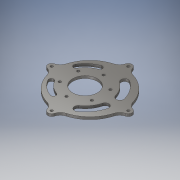
# Autodesk Inventor part: LargeBearingPlate
Saved by Autodesk Inventor 2019 (Build 230136000, 136)
## iProperties
Created: 2018-12-06
Part Number: LargeBearingPlate
Material: Aluminum 6061
Document SubType Name: Modeling
Designer: steelen
Density: 2.7 g/cm^3
Appearance: Semi-Polished
Author: steelen
Autodesk Inventor part; units mm, degrees
ref_plane "YZ Plane" through (0, 0, 0) normal (1, 0, 0) x (0, 1, 0)
ref_plane "XZ Plane" through (0, 0, 0) normal (0, 1, 0) x (-1, 0, 0)
ref_plane "XY Plane" through (0, 0, 0) normal (0, 0, 1) x (1, 0, 0)
sketch "Sketch1" plane through (0, 0, 0) normal (0, 1, 0) x (-1, 0, 0)
  circle A0 centre (12.7, 0) radius 31.75
  circle A1 centre (0, 0) radius 88.9
  circle A2 centre (0, 98.425) radius 9.525
  arc A3 (9.1574, 101.0457) -> (24.7665, 85.3805) centre (31.1351, 107.3355) ccw
  arc A4 (-24.7665, 85.3805) -> (-9.1574, 101.0457) centre (-31.1351, 107.3355) ccw
  circle A5 centre (-98.425, 0) radius 9.525
  circle A6 centre (0, -98.425) radius 9.525
  circle A7 centre (98.425, 0) radius 9.525
  arc A8 (85.3805, 24.7665) -> (101.0457, 9.1574) centre (107.3355, 31.1351) ccw
  arc A9 (24.7665, -85.3805) -> (9.1574, -101.0457) centre (31.1351, -107.3355) ccw
  arc A10 (-9.1574, -101.0457) -> (-24.7665, -85.3805) centre (-31.1351, -107.3355) ccw
  arc A11 (-85.3805, -24.7665) -> (-101.0457, -9.1574) centre (-107.3355, -31.1351) ccw
  arc A12 (-101.0457, 9.1574) -> (-85.3805, 24.7665) centre (-107.3355, 31.1351) ccw
  arc A13 (101.0457, -9.1574) -> (85.3805, -24.7665) centre (107.3355, -31.1351) ccw
  line L0 (98.425, 0) -> (88.9, 0)
  line L1 (0, 98.425) -> (0, 88.9)
  line L2 (0, -98.425) -> (0, -88.9)
  line L3 (-98.425, 0) -> (-88.9, 0)
  line L4 (12.7, 0) -> (0, 0)
  dimension "d20" = 177.8
  dimension "d0" = 63.5
  dimension "d2" = 19.05
  dimension "d3" = 22.86
  dimension "d21" = 12.7
  constraints: 27 point on circle, 13 centre point, 10 end point, 10 equal radius, 8 tangent, 3 horizontal, 3 vertical, 1 coincident, 26 other
  measures "d0" diameter of A0
  measures "d2" diameter of A2
  measures "d3" radius of A10
  measures "d21" distance of L4.start point (0, 0)
extrude "Extrusion1" add sketch "Sketch1" along normal blind 6.35
sketch "Sketch3" plane through (0, 6.35, 0) normal (0, 1, 0) x (1, 0, 0)
  circle A0 centre (-12.7, 0) radius 31.75 projected
  arc A1 (101.0457, -9.1574) -> (101.0457, 9.1574) centre (98.425, 0) ccw projected
  arc A2 (101.0457, -9.1574) -> (85.3805, -24.7665) centre (107.3355, -31.1351) ccw projected
  arc A3 (24.7665, -85.3805) -> (85.3805, -24.7665) centre (0, 0) ccw projected
  arc A4 (24.7665, -85.3805) -> (9.1574, -101.0457) centre (31.1351, -107.3355) ccw projected
  arc A5 (-9.1574, -101.0457) -> (9.1574, -101.0457) centre (0, -98.425) ccw projected
  arc A6 (-9.1574, -101.0457) -> (-24.7665, -85.3805) centre (-31.1351, -107.3355) ccw projected
  arc A7 (-85.3805, -24.7665) -> (-24.7665, -85.3805) centre (0, 0) ccw projected
  arc A8 (-85.3805, -24.7665) -> (-101.0457, -9.1574) centre (-107.3355, -31.1351) ccw projected
  arc A9 (-101.0457, 9.1574) -> (-101.0457, -9.1574) centre (-98.425, 0) ccw projected
  arc A10 (-101.0457, 9.1574) -> (-85.3805, 24.7665) centre (-107.3355, 31.1351) ccw projected
  arc A11 (-24.7665, 85.3805) -> (-85.3805, 24.7665) centre (0, 0) ccw projected
  arc A12 (-24.7665, 85.3805) -> (-9.1574, 101.0457) centre (-31.1351, 107.3355) ccw projected
  arc A13 (9.1574, 101.0457) -> (-9.1574, 101.0457) centre (0, 98.425) ccw projected
  arc A14 (9.1574, 101.0457) -> (24.7665, 85.3805) centre (31.1351, 107.3355) ccw projected
  arc A15 (85.3805, 24.7665) -> (24.7665, 85.3805) centre (0, 0) ccw projected
  arc A16 (85.3805, 24.7665) -> (101.0457, 9.1574) centre (107.3355, 31.1351) ccw projected
  constraints: 4 coincident
hole "Hole1" at (98.425, 6.35, 0) at (0, 6.35, 98.425) at (-98.425, 6.35, 0) at (0, 6.35, -98.425) direction (0, -1, 0) diameter 6.5278 depth 12.2936 tip angle 118 clearance for "Socket Head Cap Screw" size "1/4" standard "Ansi Unified Screw Threads"
sketch "Sketch8" plane through (0, 6.35, 0) normal (0, 1, 0) x (1, 0, 0)
  circle A0 centre (-12.7, 0) radius 31.75 projected
  circle A1 centre (-12.7, 0) radius 47.625
  line L0 (-12.7, 0) -> (-12.7, 47.625)
  point P0 (0, 0)
  point P1 (-53.9445, 23.8125)
  point P2 (-53.9445, -23.8125)
  point P3 (-12.7, -47.625)
  point P4 (28.5445, -23.8125)
  point P5 (28.5445, 23.8125)
  dimension "d38" = 95.25
  dimension "d41" = 360
  constraints: 2 end point, 1 coincident, 1 vertical, 1 vertical alignment, 9 other
hole "Hole3" at (-12.7, 6.35, -47.625) at (-53.9445, 6.35, -23.8125) at (-53.9445, 6.35, 23.8125) at (-12.7, 6.35, 47.625) at (28.5445, 6.35, 23.8125) at (28.5445, 6.35, -23.8125) direction (0, -1, 0) diameter 6.5278 end through all clearance for "Socket Head Cap Screw" size "1/4" standard "Ansi Unified Screw Threads"
sketch "Sketch9" plane through (0, 6.35, 0) normal (0, 1, 0) x (1, 0, 0)
  circle A0 centre (-12.7, 0) radius 31.75 projected
  circle A1 centre (-12.7, 0) radius 63.5
  circle A2 centre (-12.7, 0) radius 82.55
  arc A3 (34.6487, 67.621) -> (23.7221, 52.0162) centre (29.1854, 59.8186) ccw
  arc A4 (23.7221, -52.0162) -> (34.6487, -67.621) centre (29.1854, -59.8186) ccw
  line L0 (0, 0) -> (50.8, 0)
  line L1 (-12.7, 0) -> (29.1854, 59.8186)
  line L2 (29.1854, -59.8186) -> (-12.7, 0)
  arc A5 (67.0372, -21.3655) -> (48.6363, -16.435) centre (57.8367, -18.9003) ccw
  arc A6 (48.6363, 16.435) -> (67.0372, 21.3655) centre (57.8367, 18.9003) ccw
  line L3 (-12.7, 0) -> (57.8367, 18.9003)
  line L4 (-12.7, 0) -> (57.8367, -18.9003)
  dimension "d50" = 31.75
  dimension "d51" = 19.05
  dimension "d52" = 55
  dimension "d53" = 55
  dimension "d54" = 40
  dimension "d55" = 40
  constraints: 17 point on circle, 10 end point, 8 tangent, 6 centre point, 3 coincident, 1 horizontal
  measures "d50" radial gap between concentric circles of A1 A0
  measures "d51" radial gap between concentric circles of A1 A2
  measures "d52" angle of L2 L0
  measures "d53" angle of L0 L1
  measures "d54" angle of L1 L3
  measures "d55" angle of L2 L4
extrude "Extrusion3" cut sketch "Sketch9" against normal blind 25.4 contours A1 A3 A2 A6 | A5 A2 A4 A1
sketch "Sketch10" plane through (0, 6.35, 0) normal (0, 1, 0) x (1, 0, 0)
  circle A0 centre (-98.425, 0) radius 3.2639
  line L0 (-12.7, 0) -> (-98.425, 0)
  arc A1 (-32.2465, 53.7034) -> (-62.1934, 28.575) centre (-12.7, 0) ccw
  arc A2 (-73.1919, 34.925) -> (-62.1934, 28.575) centre (-67.6926, 31.75) ccw
  arc A3 (-32.2465, 53.7034) -> (-36.5901, 65.6375) centre (-34.4183, 59.6705) ccw
  arc A4 (-36.5901, 65.6375) -> (-73.1919, 34.925) centre (-12.7, 0) ccw
  circle A5 centre (-98.425, 0) radius 3.2639 projected
  circle A6 centre (-12.7, 0) radius 31.75 projected
  arc A7 (-62.1934, -28.575) -> (-32.2465, -53.7034) centre (-12.7, 0) ccw
  arc A8 (-62.1934, -28.575) -> (-73.1919, -34.925) centre (-67.6926, -31.75) ccw
  arc A9 (-36.5901, -65.6375) -> (-32.2465, -53.7034) centre (-34.4183, -59.6705) ccw
  arc A10 (-73.1919, -34.925) -> (-36.5901, -65.6375) centre (-12.7, 0) ccw
  circle A11 centre (-12.7, 0) radius 31.75
  dimension "d58" = 114.3
  dimension "d59" = 12.7
  dimension "d60" = 70
  dimension "d61" = 30
  constraints: 16 point on circle, 10 centre point, 6 symmetric about line, 4 tangent, 3 coincident, 3 end point, 2 equal radius, 1 concentric, 1 horizontal, 5 other
  measures "d58" diameter of A1
  measures "d59" diameter of A3
extrude "Extrusion4" cut sketch "Sketch10" against normal blind 25.4 contours A1 A2 A4 A3 | A7 A9 A10 A8
body "Solid1"
